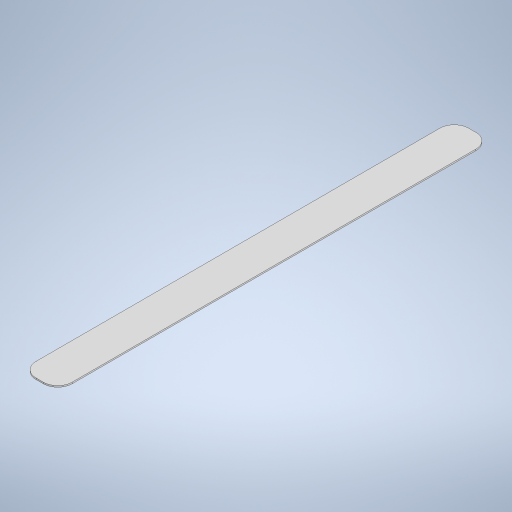
# Autodesk Inventor part: popsicle stick
Saved by Autodesk Inventor 2023 (Build 270158000, 158)
## iProperties
Created: 2023-01-20
Part Number: popsicle stick
Material: Generic
Document SubType Name: Modeling
Designer: kavya
Density: 1 g/cm^3
Appearance: Default
Author: kavya
Autodesk Inventor part; units mm, degrees
ref_plane "YZ Plane" through (0, 0, 0) normal (1, 0, 0) x (0, 1, 0)
ref_plane "XZ Plane" through (0, 0, 0) normal (0, 1, 0) x (-1, 0, 0)
ref_plane "XY Plane" through (0, 0, 0) normal (0, 0, 1) x (1, 0, 0)
sketch "Sketch1" plane through (0, 0, 0) normal (0, 1, 0) x (-1, 0, 0)
  line L0 (10, 0) -> (15, 0)
  line L1 (25, -10) -> (25, -290)
  line L2 (15, -300) -> (10, -300)
  line L3 (0, -290) -> (0, -10)
  arc A0 (25, -2) -> (23, 0) centre (23, -2) ccw
  arc A1 (25, -10) -> (15, 0) centre (15, -10) ccw
  arc A2 (10, 0) -> (0, -10) centre (10, -10) ccw
  arc A3 (0, -290) -> (10, -300) centre (10, -290) ccw
  arc A4 (15, -300) -> (25, -290) centre (15, -290) ccw
  point P0 (0, 0)
  point P1 (25, -300)
  point P2 (25, 0)
  point P3 (0, -300)
  dimension "d0" = 25
  dimension "d1" = 300
  dimension "d2" = 2
  dimension "d3" = 10
  constraints: 10 point on circle, 10 point on line, 10 tangent, 8 end point, 5 centre point, 3 equal radius, 2 parallel, 1 horizontal, 1 perpendicular
  measures "d0" distance of point (25, -300) point (0, -300)
  measures "d1" distance of point (25, 0) point (25, -300)
  measures "d2" radius of A0
  measures "d3" radius of A1
extrude "Extrusion1" add sketch "Sketch1" along normal blind 1
body "Solid1"
